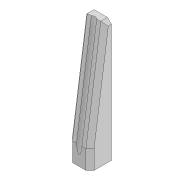
# Autodesk Inventor part: GB-stand
Saved by Autodesk Inventor 2020 (Build 240168000, 168)
## iProperties
Created: 2021-07-13
Part Number: GB-stand
Material: Generic
Document SubType Name: Modeling
Designer: Aidan Lee
Density: 1 g/cm^3
Appearance: Default
Author: Aidan Lee
Autodesk Inventor part; units mm, degrees
ref_plane "YZ Plane" through (0, 0, 0) normal (1, 0, 0) x (0, 1, 0)
ref_plane "XZ Plane" through (0, 0, 0) normal (0, 1, 0) x (-1, 0, 0)
sketch "Sketch1" plane through (0, 0, 0) normal (0, 0, 1) x (1, 0, 0)
  circle A0 centre (0, 165) radius 11
  line L0 (-11, 0) -> (-5, 0) construction
  line L1 (-5, 0) -> (-5, 24.6936) construction
  line L2 (-5, 24.6936) -> (-11, 24.6936) construction
  line L3 (-11, 24.6936) -> (-11, 0) construction
  line L4 (0, 0) -> (0, -33.6453) construction
  line L5 (11, 0) -> (5, 0) construction
  line L6 (5, 0) -> (5, 24.6936) construction
  line L7 (5, 24.6936) -> (11, 24.6936) construction
  line L8 (11, 24.6936) -> (11, 0) construction
  line L9 (16, 0) -> (-16, 0) construction
  line L10 (-16, 0) -> (-16, 181) construction
  line L11 (-16, 181) -> (16, 181) construction
  line L12 (16, 181) -> (16, 0) construction
  line L13 (-11, 168.4627) -> (-11, 161.5373) construction
  line L14 (-3.4627, 176) -> (3.4627, 176) construction
  point P0 (0, 0)
  point P1 (-11, 165)
  point P2 (0, 176)
  dimension "d0" = 22
  dimension "d1" = 165
  dimension "d2" = 6
  dimension "d3" = 10
  dimension "d4" = 5
  dimension "d8" = 5
  dimension "d9" = 5
  dimension "d10" = 32
  constraints: 30 end point, 4 parallel, 4 symmetric about line, 3 horizontal, 3 midpoint, 3 perpendicular, 2 point on circle, 2 vertical, 2 vertical alignment, 1 centre point, 1 coincident, 1 horizontal alignment
  measures "d0" diameter of A0
  measures "d1" distance of L4.start A0.centre
  measures "d2" distance of L1.end L2.end
  measures "d3" distance between parallel lines of L1 L6
  measures "d4" distance between parallel lines of L10 L3
  measures "d8" distance between parallel lines of L10 L13
  measures "d9" distance between parallel lines of L11 L14
  measures "d10" distance of L10.end L11.end
sketch "Sketch2" plane through (0, 0, 0) normal (1, 0, 0) x (0, 1, 0)
  line L0 (0, 0) -> (181, 0)
  line L1 (181, 0) -> (181, 32) construction
  line L2 (181, 32) -> (0, 32) construction
  line L3 (0, 32) -> (0, 0)
  line L4 (0, 27) -> (25, 27)
  line L5 (25, 27) -> (25, 21)
  line L6 (25, 21) -> (0, 21)
  line L7 (0, 21) -> (0, 27)
  line L8 (25, 11) -> (0, 11)
  line L9 (0, 11) -> (0, 5)
  line L10 (0, 5) -> (25, 5)
  line L11 (25, 5) -> (25, 11)
  line L12 (0, 32) -> (28, 32)
  line L13 (176, 0) -> (154, 0) projected
  line L14 (176, 0) -> (154, 0) construction
  line L15 (154, 0) -> (154, 7) construction
  line L16 (154, 7) -> (176, 7) construction
  line L17 (176, 7) -> (176, 0) construction
  line L18 (181, 0) -> (181, 10)
  line L19 (181, 10) -> (28, 32)
  dimension "d7" = 32
  dimension "d11" = 6
  dimension "d12" = 10
  dimension "d13" = 5
  dimension "d14" = 25
  dimension "d15" = 7
  dimension "d16" = 3
  dimension "d17" = 3
  constraints: 38 end point, 8 parallel, 5 point on line, 4 horizontal, 4 perpendicular, 1 coincident, 1 collinear
  measures "d7" distance of L2.end L0.start
  measures "d11" distance of L4.end L5.end
  measures "d12" distance between parallel lines of L8 L6
  measures "d13" distance between parallel lines of L2 L4
  measures "d14" distance between parallel lines of L3 L5
  measures "d15" distance of L13.end L15.end
  measures "d16" distance from line of L18.end L16
  measures "d17" distance from line of L12.end L5
extrude "Extrusion1" add sketch "Sketch2" along normal mid plane 32
chamfer "Chamfer1" distance 6 angle 45 6 edges at (-16, 104.5, 21) (-16, 14, 32) (16, 14, 32) (16, 104.5, 21) (-16, 181, 5) (16, 181, 5)
extrude "Extrusion2" cut sketch "Sketch1" along normal blind 7
sketch "Sketch3" plane through (-10, 181, 10) normal (0, 0.1423, 0.9898) x (1, 0, 0)
  line L0 (0, 0) -> (20, 0) projected
  line L1 (10, 0) -> (10, -154.5736)
  line L2 (0, -154.5736) -> (20, -154.5736) projected
  point P0 (10, -177.7341)
  constraints: 2 end point, 2 midpoint
ref_plane "Work Plane1" through (0, 28, 32) normal (0, -0.9898, 0.1423) x (1, 0, 0)
sketch "Sketch4" plane through (0, 28, 32) normal (0, -0.9898, 0.1423) x (1, 0, 0)
  circle A0 centre (0, 3.4008) radius 5.2132
  point P0 (0, -35.6594)
  constraints: 1 centre point
extrude "Extrusion3" cut sketch "Sketch4" against normal through all both and the other way through all
sketch "Sketch5" plane through (-16, 0, 0) normal (0, -1, 0) x (1, 0, 0)
  circle A0 centre (8, 8) radius 3
  circle A1 centre (24, 8) radius 3
  circle A2 centre (16, 24) radius 3
  line L0 (32, 0) -> (0, 0) projected
  line L1 (24, 8) -> (8, 8) construction
  point P0 (16, 0)
  point P1 (16, 0)
  point P2 (16, 8)
  point P3 (16, 0)
  dimension "d27" = 6
  dimension "d28" = 16
  dimension "d29" = 8
  dimension "d30" = 16
  constraints: 3 centre point, 3 midpoint, 2 end point, 2 equal radius, 2 vertical alignment, 1 horizontal, 1 horizontal alignment
  measures "d27" diameter of A2
  measures "d28" distance of L1.start L1.end
  measures "d29" distance from line of L0 L1.end
  measures "d30" distance from line of A2.centre L1
extrude "Extrusion4" cut sketch "Sketch5" against normal blind 32
thread "Thread1" size "M6x1" class "6H" standard "ANSI Metric M Profile" full length
thread "Thread2" size "M6x1" class "6H" standard "ANSI Metric M Profile" full length
thread "Thread3" size "M6x1" class "6H" standard "ANSI Metric M Profile" full length
equation "\"d4\" = 0.5 * d3"
equation "\"d18\" = d10"
equation "\"d30\" = d28"
equation "\"d31\" = d10"
body "Solid1"
